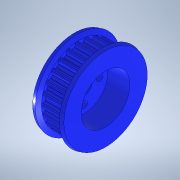
# Autodesk Inventor part: TimingPulley_S5M_MechaLock_1
Saved by Autodesk Inventor 2022 (Build 260153000, 153)
## iProperties
Category: PARTsolutions
Company: MISUMI
Part Number: TimingPulley_S5M_MechaLock_1
Material: ABS プラスチック
Catalog Web Link: www.cadenas.de
Description: HTPA__S5M100, HTPA__S5M150, HTPA__S5M250, HTPB__S5M100, HTPB__S5M150, HTPB__S5M250, HTPK__S5M100, HTPK__S5M150, HTPK__S5M250, HTPN__S5M100, HTPN__S5M150, HTPN__S5M250, HTPT__S5M100, HTPT__S5M150, HTPT__S5M250, HTPM__S5M100, HTPM__S5M150, HTPM__S5M250, HTPP__S5M100, HTPP__S5M150, HTPP__S5M250, HTPS__S5M100, HTPS__S5M150_body-High Torque Timing Pulleys S5M Type
Vendor: MISUMI
Document SubType Name: Modeling
Designer: partserver
Manufacturer: MISUMI
Mass: 10.4108 g
Surface Area: 49.6808 cm^2
Volume: 10.4108 cm^3
Density: 1.06 g/cm^3
Appearance: 青 - 壁塗料 - 光沢
PSOL_IDENT_0: {$CADENAS_DATA\23d-libs\misumi\metric\51_timing_pulleys\htpb_s5m\htpb_s5m.prj},732 {VTYP=3D},{NB=HTP
PSOL_IDENT_1: A20S5M100-A-H8_b},{LINA=HTPA20S5M100-A-H8},{NN=HTPA__S5M100, HTPA__S5M150, HTPA__S5M250, HTPB__S5M10
PSOL_IDENT_2: 0, HTPB__S5M150, HTPB__S5M250, HTPK__S5M100, HTPK__S5M150, HTPK__S5M250, HTPN__S5M100, HTPN__S5M150,
PSOL_IDENT_3: HTPN__S5M250, HTPT__S5M100, HTPT__S5M150, HTPT__S5M250, HTPM__S5M100, HTPM__S5M150, HTPM__S5M250, H
PSOL_IDENT_4: TPP__S5M100, HTPP__S5M150, HTPP__S5M250, HTPS__S5M100, HTPS__S5M150_body},{DATE=17.01.2019 01:25:31}
PSOL_IDENT_5: ,{GEOMDATE=28.12.2018 04:09:27},{VERSION=},{LINEID=70},{WBVAR=MATP,ST,TNW,PS,SBS,DD,Z,J,Q,R,S,T,ALT1
PSOL_IDENT_6: ,ALT2,M,QSC,QFC,QTC,ALT3,K,KSC,KFC,KTC,ALT4,ZM,ZSC,ZFC,ZTC,ALT5,ALT6,ALT7,FC,ALT8,SRG,ALT9,BTC,TL,AL
PSOL_IDENT_7: T10,TPC,ALT11,BC,ALT12,SLH},{WBNUMERIC=DD,Z,J,Q,R,S,T,QSC,QFC,QTC,K,KSC,KFC,KTC,ZSC,ZFC,ZTC,FC,SRG,B
PSOL_IDENT_8: TC,TL,BC,SLH}  {NB=HTPA20S5M100-A-H8_b},{LINA=HTPA20S5M100-A-H8},{KT=DUMMY},{PN=HTPA20S5M100-A-H8},{
PSOL_IDENT_9: TYPE=HTPA},{MATP=A2017},{MATPALG= 'A2017','Aluminum Alloy 2000 series','S45C','1045 Carbon Steel Equ
PSOL_IDENT_10: ivalent','SUS304','SUS304' },{ST=CA},{STALG= 'CA','Clear Anodize','BA','Black Anodize','HAT','Hard C
PSOL_IDENT_11: lear Anodize','ENP','Electroless Nickel Plating' },{NT=20},{TNW=S5M100},{TNWALG= 'S5M100','S5M150','
PSOL_IDENT_12: S5M250' },{BW=10},{PS=A},{PSALG= 'A','B' },{SBS=H},{SBSALG= 'H','Round Hole','P','Round Hole + Tap','
PSOL_IDENT_13: N','New JIS Keywayed Bore + Tap (Standard)','NK','New JIS Keywayed Bore + Tap (width 4.0mm, height 1
PSOL_IDENT_14: .8mm)','C','Old JIS Keywayed Bore + Tap','V','Stepped Hole','Y','Both Ends Stepped Hole','WB','Doubl
PSOL_IDENT_15: e Stepped Hole' },{DD=8.00},{DDALG=[6:6/1],6.35,[7:12/1],12.7,[13:20/1]},{DDHA=[6:6/1],6.35,[7:12/1]
PSOL_IDENT_16: ,12.7,[13:20/1]},{DDPA=[6:6/1],6.35,[7:12/1],12.7,[13:16/1]},{DDNA=[8:8/1],[10:16/1]},{DDCA=[10,12,1
PSOL_IDENT_17: 5,16]},{DDVA=[6:6/1],6.35,[7:12/1],12.7,[13:18/1]},{DDY=[6:18/1]},{DDWB=[6:16/1]},{DDHB=},{DDPB=},{D
PSOL_IDENT_18: DNB=},{DDNK=[10:10/1]},{DDCB=},{DDVFB=},{Z=0},{ZALG=[0]},{ZMIN=10.000},{ZAMAX=20.000},{ZBMAX=0.000},
PSOL_IDENT_19: {DDZ=8.000},{J=0.0},{JALG=[0]},{JMIN=2.000},{JMAX=14.000},{JPN=},{Q=0},{QALG=[0]},{QRMIN=10.000},{QR
PSOL_IDENT_20: MAX=20.000},{WBQMIN=12.000},{R=0},{RALG=[0]},{WBRMAX=-2.000},{S=0.0},{SALG=[0]},{SMAX=10.000},{T=0.0
PSOL_IDENT_21: },{TALG=[0]},{TMAX=13.000},{SBSPN=-H8},{A=11},{W=16},{L=0},{PD=31.83},{OD=30.87},{D=0},{DALG=19.000}
PSOL_IDENT_22: ,{DE=24.000},{F=36},{E=24},{TT=1.6},{BBK=0.000},{TTK=0.000},{ALT1=},{ALT1ALG= '','Not applicable' },
PSOL_IDENT_23: {ANG=126.000},{ALT1PN=},{ALT2=},{ALT2ALG= '','w/o Side Tapped Hole','QSC','with QSC (6 Places Side T
PSOL_IDENT_24: apped Hole)','QFC','with QFC (4 Places Side Tapped Hole)','QTC','with QTC (3 Places Side Tapped Hole
PSOL_IDENT_25: )' },{M=N/A},{MALG= 'N/A' },{MFTALG= 'N/A' },{MSALG= 'N/A' },{M3D=0.000},{KDML=0.000},{ML=0.000},{MU
PSOL_IDENT_26: L=0.000},{PITCH=0.000},{QSC=0.0},{QSCALG=0},{QFC=0.0},{QFCALG=0},{QTC=0.0},{QTCALG=0},{QPCDMIN=0.000
PSOL_IDENT_27: },{QPCDMINALG=0.000},{QPCDMAX=20.000},{ALT2PN=},{TAP=0.000},{ALT3=},{ALT3ALG= '','w/o Side Through H
PSOL_IDENT_28: ole','KSC','with KSC (6 Places Side Through Hole)','KFC','with KFC (4 Places Side Through Hole)','KT
PSOL_IDENT_29: C','with KTC (3 Places Side Through Hole)' },{K=0.0},{KALG=0},{KMIN=4.000},{KFTMAX=4.000},{KSMAX=4.0
PSOL_IDENT_30: 00},{KSC=0.0},{KSCALG=0},{KFC=0.0},{KFCALG=0},{KTC=0.0},{KTCALG=0},{KSCMIN=12.000},{KSCMINALG=12},{K
PSOL_IDENT_31: PCDMIN=12.000},{KPCDMINALG=12},{KPCDMAX=20.000},{ALT3PN=},{ALT4=},{ALT4ALG= '','Not applicable' },{A
PSOL_IDENT_32: LT4MIN=18.500},{ALT4MAX=13.500},{ZM=N/A},{ZMALG= 'N/A' },{ZMFTALG= 'N/A' },{ZMSALG= 'N/A' },{ZMDD1=0
PSOL_IDENT_33: .0},{ZMDD2=0.0},{ZMHH=0.0},{ZSC=0.0},{ZSCALG=[0]},{ZFC=0.0},{ZFCALG=[0]},{ZTC=0.0},{ZTCALG=[0]},{ZPC
PSOL_IDENT_34: DMIN=0.000},{ZPCDMINALG=0.000},{ZPCDMAX=20.000},{ALT4PN=},{ALT5=},{ALT5ALG= '','w/o Flange not Attac
PSOL_IDENT_35: hed','NFC','with NFC (Flange not Attached)' },{ALT5PN=},{ALT6=},{ALT6ALG= '','w/o Flange Attached on
PSOL_IDENT_36: One Side Only','RFC','with RFC (Flange Attached on The Boss Side Only)','LFC','with LFC (Flange Att
PSOL_IDENT_37: ached on The Opposite Side Only)' },{ALT6PN=},{ALT7=},{ALT7ALG= '','w/o FC (Flange Cut)','FC','with
PSOL_IDENT_38: FC (Flange Cut)' },{FC=0.0},{FCALG=0},{FCMIN=32.0},{FCMAX=34.0},{ALT7PN=},{ALT8=},{ALT8ALG= '','Not
PSOL_IDENT_39: applicable' },{ALT8ALGALG=20.000},{ALT8DD2=0.000},{ALT8MM=0.000},{ALT8NN=0.000},{QC=0.000},{KC=0.000
PSOL_IDENT_40: },{ZC=0.000},{SRG=0.0},{SRGALG=[0]},{SRGMAX=0.000},{DD2=0.0},{MM=0.00},{NN=0.00},{ALT8PN=},{ALT9=},{
PSOL_IDENT_41: ALT9ALG= '','w/o BTC (Taper for Bearing Holder)','BTC','with BTC (Taper for Bearing Holder)' },{BTC9=
PSOL_IDENT_42: 9.000},{TL9=1.000},{BTC=0},{BTCALG=[0]},{TL=0.0},{TLALG=0},{TLMIN=1.000},{TLMAX=-16.500},{BTCL=0},{B
PSOL_IDENT_43: TCD=0},{ALT9PN=},{WLBCTL=16.000},{ALT10=},{ALT10ALG= '','Not applicable' },{TPC=N/A},{TPCALG= 'N/A'
PSOL_IDENT_44: },{TPCM=4.000},{ALT10PN=},{ALT11=},{ALT11ALG= '','Not applicable' },{BC=0.0},{BCALG=0},{BCMIN=3.000}
PSOL_IDENT_45: ,{BCMAX=-16.500},{M1WBC=8.000},{ALT11PN=},{KTT=11.435},{ALT12=},{ALT12ALG= '','Not applicable' },{SL
PSOL_IDENT_46: H=0},{SLHALG=[0]},{ALT12PN=},{AC=-},{M1=4.000},{M1L=3.000}
NB: HTPA20S5M100-A-H8_b
NN: 0
NT: 20
NBSYN: $PN._b
LINA: HTPA20S5M100-A-H8
CATALOG: Misumi
PN: HTPA20S5M100-A-H8
MATP: Aluminum Alloy 2000 series
ST: Clear Anodize
TNW: S5M100
BW: 10
PS: A
SBS: Round Hole
DD: 8
Z: 0
J: 0
Q: 0
R: 0
S: 0
T: 0
A: 11
W: 16
L: 0
PD: 31.83
OD: 30.87
D: 0
F: 36
E: 24
TT: 1.6
ALT1: Not applicable
ALT2: w/o Side Tapped Hole
M: N/A
QSC: 0
QFC: 0
QTC: 0
ALT3: w/o Side Through Hole
K: 0
KSC: 0
KFC: 0
KTC: 0
ALT4: Not applicable
ZM: N/A
ZMDD1: 0
ZMDD2: 0
ZMHH: 0
ZSC: 0
ZFC: 0
ZTC: 0
ALT5: w/o Flange not Attached
ALT6: w/o Flange Attached on One Side Only
ALT7: w/o FC (Flange Cut)
FC: 0
ALT8: Not applicable
SRG: 0
DD2: 0
MM: 0
ALT9: w/o BTC (Taper for Bearing Holder)
BTC: 0
TL: 0
BTCL: 0
BTCD: 0
ALT10: Not applicable
TPC: N/A
ALT11: Not applicable
BC: 0
ALT12: Not applicable
SLH: 0
AC: -
SUPPLIER: MISUMI
ARTICLENO: HTPA20S5M100-A-H8_b
BOMINFO: HTPA20S5M100-A-H8
CREATOR: CADENAS GmbH
d128: 25.000 mm
歯数: 25.000 ul
歯幅: 11.000 mm
穴径: 8.300 mm
穴間隔: 15.800 mm
Title: HTPA20S5M100-A-H8
Author: Cadenas PARTsolutions
Comments: High Torque Timing Pulleys S5M Type
Autodesk Inventor part; units mm, degrees
note: some values were not read from the file. Chosen so that the rebuilt part matches the saved one: pattern direction of "Circular Pattern1".
ref_plane "YZ Plane" through (0, 0, 0) normal (1, 0, 0) x (0, 1, 0)
ref_plane "XZ Plane" through (0, 0, 0) normal (0, 1, 0) x (-1, 0, 0)
sketch "_____2" plane through (0, 0, 0) normal (0, 0, 1) x (1, 0, 0)
  line L0 (0, 0) -> (0, 13.5)
  line L1 (0, 13.5) -> (0.9, 13.5)
  line L2 (0.9, 13.5) -> (0.9, 19.2037)
  line L3 (0.9, 19.2037) -> (0.2846, 21.5003)
  line L4 (0.2846, 21.5003) -> (1.8301, 21.9144)
  line L5 (1.8301, 21.9144) -> (2.5, 19.4144)
  line L6 (2.5, 19.4144) -> (13.5, 19.4144)
  line L7 (13.5, 19.4144) -> (14.1699, 21.9144)
  line L8 (14.1699, 21.9144) -> (15.7154, 21.5003)
  line L9 (15.7154, 21.5003) -> (15.1, 19.2037)
  line L10 (15.1, 19.2037) -> (15.1, 13.5)
  line L11 (15.1, 13.5) -> (16, 13.5)
  line L12 (16, 13.5) -> (16, 0)
  line L13 (16, 0) -> (0, 0)
  line L14 (8, 19.4144) -> (8, 0) construction
  line L15 (0, 13.5) -> (0, 21.424)
  line L16 (0, 21.424) -> (0.2846, 21.5003)
  line L17 (16, 13.5) -> (16, 21.424)
  line L18 (16, 21.424) -> (15.7154, 21.5003)
  line L19 (13.5, 19.4144) -> (13.5, 0)
  line L20 (2.5, 19.4144) -> (2.5, 0)
  dimension "d40" = 19.4144
  dimension "d41" = 16
  dimension "d42" = 11
  dimension "d43" = 105
  dimension "d53" = 1.6
  dimension "d54" = 13.5
  dimension "d55" = 0.9
  dimension "d56" = 2.5
  constraints: 42 end point, 10 perpendicular, 3 vertical, 2 collinear, 2 midpoint, 2 point on line, 1 coincident, 1 horizontal, 1 parallel, 1 vertical alignment, 5 other
  measures "d40" distance between parallel lines of L13 L6
  measures "d41" distance of L12.end L0.start
  measures "d42" distance of L5.end L6.end
  measures "d43" angle of L6 L5
  measures "d53" distance of L3.end L4.end
  measures "d54" distance of L0.start L0.end
  measures "d55" distance of L0.end L1.end
  measures "d56" vertical distance of L5.end L4.end
revolve "Revolution1" add sketch "_____2" angle 360 about axis through (16, 0, 0) along (1, 0, 0)
sketch "_____6" plane through (2.5, 0, 0) normal (1, 0, 0) x (0, 0, -1)
  arc A0 (-1.5181, 18.9076) -> (-2.1055, 19.2999) centre (-2.0459, 18.7531) ccw
  arc A1 (-1.5181, 18.9076) -> (-0.8816, 17.7202) centre (1.625, 19.8279) ccw
  arc A2 (-0.8816, 17.7202) -> (-0.6806, 17.6312) centre (-0.6903, 17.881) ccw
  arc A3 (0.6806, 17.6312) -> (-0.6806, 17.6312) centre (0, 0) ccw
  arc A4 (0.6806, 17.6312) -> (0.8816, 17.7202) centre (0.6903, 17.881) ccw
  arc A5 (0.8816, 17.7202) -> (1.5181, 18.9076) centre (-1.625, 19.8279) ccw
  arc A6 (2.1055, 19.2999) -> (1.5181, 18.9076) centre (2.0459, 18.7531) ccw
  line L0 (2.1055, 19.2999) -> (2.1055, 19.7826)
  arc A7 (2.1055, 19.7826) -> (-2.1055, 19.7826) centre (0, 0) ccw
  line L1 (-2.1055, 19.7826) -> (-2.1055, 19.2999)
  line L2 (0, 0) -> (0, 19.8944)
  arc A8 (2.1055, 19.2999) -> (-2.1055, 19.2999) centre (0, 0) ccw construction
  dimension "d44" = 0.55
  dimension "d45" = 3.275
  dimension "d46" = 0.25
  dimension "d47" = 2.25
  dimension "d49" = 19.8944
  dimension "d50" = 0.48
  dimension "d52" = 3.25
  constraints: 20 point on circle, 9 centre point, 7 tangent, 6 end point, 3 coincident, 3 equal radius, 2 vertical, 4 other
  measures "d44" radius of A6
  measures "d45" radius of A5
  measures "d46" radius of A4
  measures "d47" radial gap between concentric circles of A7 A3
  measures "d49" distance of L2.start L2.end
  measures "d50" radial gap between concentric circles of A7 A8
  measures "d52" distance of A1.centre A5.centre
extrude "Extrusion1" cut sketch "_____6" along normal blind 11
pattern_circular "Circular Pattern1" count 25 over 360 about axis through (8, 0, 0) along (1, 0, 0) of "Extrusion1"
sketch "スケッチ21" plane through (0, 0, 0) normal (-1, 0, 0) x (0, 0, 1)
  circle A0 centre (0, 0) radius 12.5
  dimension "d128" = 25
  constraints: 1 centre point, 1 coincident
  measures "d128" diameter of A0
ref_plane "作業平面2" through (11, 0, 0) normal (1, 0, 0) x (0, 0, -1)
sketch "スケッチ22" plane through (11, 0, 0) normal (1, 0, 0) x (0, 0, -1)
  circle A0 centre (0, 0) radius 12.0188
  dimension "d130" = 24.0376
  constraints: 1 centre point, 1 coincident
  measures "d130" diameter of A0
loft "ロフト3" cut profiles "スケッチ21", "スケッチ22"
sketch "スケッチ23" plane through (16, 0, 0) normal (1, 0, 0) x (0, 0, -1)
  point P0 (0, 0)
  point P1 (0, 0)
  constraints: 1 coincident
hole "穴7" at (16, 0, 0) direction (-1, 0, 0) diameter 8.3 end through all
sketch "スケッチ24" plane through (16, 0, 0) normal (1, 0, 0) x (0, 0, -1)
  point P0 (0, 0)
  point P1 (0, 8)
  point P2 (-8, 0)
  point P3 (0, -8)
  point P4 (8, 0)
  dimension "d142" = 8
  dimension "d145" = 360
  constraints: 1 vertical alignment, 5 other
  measures "d142" distance of point (0, 0) point (0, 8)
hole "穴8" at (16, 8, 0) at (16, 0, 8) at (16, -8, 0) at (16, 0, -8) direction (-1, 0, 0) diameter 3.4 end through all
sketch "スケッチ25" plane through (16, 0, 0) normal (1, 0, 0) x (0, 0, -1)
  line L0 (14.453, -10.5145) -> (8.4229, -16.5446) construction
  line L1 (8.4229, -16.5446) -> (4.1903, -12.3121) construction
  line L2 (4.1903, -12.3121) -> (10.2205, -6.2819) construction
  line L3 (10.2205, -6.2819) -> (14.453, -10.5145) construction
  line L4 (0, 0) -> (-21.424, 0) construction
  circle A0 centre (0, 0) radius 21.424 construction
  line L5 (7.5565, -8.8651) -> (11.5483, -4.8733)
  line L6 (11.5483, -4.8733) -> (12.16, -5.485)
  spline S0 degree 2 poles (12.16, -5.485) (11.9992, -6.1841) (11.7335, -7.4495) (11.6357, -8.0856) knots 0 0 0 1 2 2 2
  spline S1 degree 2 poles (11.6357, -8.0856) (11.4364, -9.3685) (11.5483, -10.5569) (11.8943, -10.9029) knots 0 0 0 1 2 2 2
  spline S2 degree 2 poles (11.8943, -10.9029) (12.0761, -11.0847) (12.52, -11.1861) (12.7542, -11.1266) knots 0 0 0 1 2 2 2
  spline S3 degree 2 poles (12.7542, -11.1266) (12.9919, -11.0637) (13.4812, -10.7491) (13.7189, -10.5115) knots 0 0 0 1 2 2 2
  spline S4 degree 2 poles (13.7189, -10.5115) (13.9496, -10.2808) (14.3481, -9.7285) (14.5054, -9.4523) knots 0 0 0 1 2 2 2
  spline S5 degree 2 poles (14.5054, -9.4523) (14.6382, -9.2216) (14.8375, -8.7428) (14.8934, -8.589) knots 0 0 0 1 2 2 2
  line L7 (14.8934, -8.589) -> (14.9423, -8.54)
  line L8 (14.9423, -8.54) -> (15.5575, -9.1552)
  spline S6 degree 2 poles (15.5575, -9.1552) (15.3758, -9.5118) (14.5858, -10.6443) (14.1559, -11.0742) knots 0 0 0 1 2 2 2
  spline S7 degree 2 poles (14.1559, -11.0742) (13.254, -11.976) (11.5902, -12.3605) (11.0449, -11.8152) knots 0 0 0 1 2 2 2
  spline S8 degree 2 poles (11.0449, -11.8152) (10.7898, -11.5601) (10.5416, -10.9554) (10.5171, -10.6163) knots 0 0 0 1 2 2 2
  spline S9 degree 2 poles (10.5171, -10.6163) (10.4892, -10.2668) (10.5695, -9.4454) (10.643, -9.0154) knots 0 0 0 1 2 2 2
  spline S10 degree 2 poles (10.643, -9.0154) (10.7548, -8.3093) (11.1218, -6.67) (11.2372, -6.1841) knots 0 0 0 1 2 2 2
  line L9 (11.2372, -6.1841) -> (8.0563, -9.365)
  line L10 (8.0563, -9.365) -> (7.5565, -8.8651)
  spline S11 degree 2 poles (4.1415, -15.0206) (3.8304, -14.7095) (3.5997, -13.8775) (3.6731, -13.4127) knots 0 0 0 1 2 2 2
  spline S12 degree 2 poles (3.6731, -13.4127) (3.75, -12.9443) (4.3372, -11.9026) (4.8406, -11.3993) knots 0 0 0 1 2 2 2
  spline S13 degree 2 poles (4.8406, -11.3993) (5.3054, -10.9344) (6.3401, -10.1724) (6.7805, -9.9487) knots 0 0 0 1 2 2 2
  line L11 (6.7805, -9.9487) -> (7.3922, -10.5604)
  line L12 (7.3922, -10.5604) -> (7.3328, -10.6198)
  spline S14 degree 2 poles (7.3328, -10.6198) (7.1825, -10.6722) (6.6826, -10.9204) (6.3995, -11.0917) knots 0 0 0 1 2 2 2
  spline S15 degree 2 poles (6.3995, -11.0917) (6.0849, -11.2874) (5.5921, -11.6475) (5.3264, -11.9131) knots 0 0 0 1 2 2 2
  spline S16 degree 2 poles (5.3264, -11.9131) (5.0643, -12.1753) (4.6972, -12.794) (4.6553, -13.1086) knots 0 0 0 1 2 2 2
  spline S17 degree 2 poles (4.6553, -13.1086) (4.6238, -13.3987) (4.7951, -13.9125) (5.0258, -14.1432) knots 0 0 0 1 2 2 2
  spline S18 degree 2 poles (5.0258, -14.1432) (5.2565, -14.3739) (5.7354, -14.4823) (6.0115, -14.4019) knots 0 0 0 1 2 2 2
  spline S19 degree 2 poles (6.0115, -14.4019) (6.3086, -14.3215) (6.9413, -13.8706) (7.2769, -13.535) knots 0 0 0 1 2 2 2
  spline S20 degree 2 poles (7.2769, -13.535) (7.6299, -13.182) (8.2696, -12.3955) (8.4513, -12.1508) knots 0 0 0 1 2 2 2
  line L13 (8.4513, -12.1508) -> (10.6744, -14.3739)
  line L14 (10.6744, -14.3739) -> (7.1231, -17.9252)
  line L15 (7.1231, -17.9252) -> (6.6162, -17.4184)
  line L16 (6.6162, -17.4184) -> (9.3322, -14.7025)
  line L17 (9.3322, -14.7025) -> (8.1822, -13.5525)
  spline S21 degree 2 poles (8.1822, -13.5525) (8.0389, -13.7237) (7.7452, -14.0383) (7.6194, -14.1642) knots 0 0 0 1 2 2 2
  spline S22 degree 2 poles (7.6194, -14.1642) (7.1231, -14.6605) (6.3261, -15.2408) (5.8472, -15.3981) knots 0 0 0 1 2 2 2
  spline S23 degree 2 poles (5.8472, -15.3981) (5.3649, -15.5588) (4.533, -15.412) (4.1415, -15.0206) knots 0 0 0 1 2 2 2
  point P0 (12.3368, -8.3982)
  point P1 (18.7618, -10.3431)
  dimension "歯数" = 25
  dimension "d154" = 45
  dimension "d155" = 21.424
  dimension "d156" = 14.924
  constraints: 2 end point, 2 point on circle, 1 horizontal, 1 midpoint, 2 other
  measures "d154" angle of L4 L0
  measures "d155" distance of A0.end L4.start
  measures "d156" distance of point (12.337, -8.398) A0.centre
extrude "押し出し11" cut sketch "スケッチ25" against normal blind 1
equation "\"d42\" = 歯幅"
equation "\"d49\" = 0.795775 * 歯数"
equation "\"d8\" = 歯幅"
equation "\"d135\" = 穴径"
equation "\"歯数\" = 25"
equation "\"歯幅\" = 11"
equation "\"穴径\" = 8.3"
body "Solid1"
